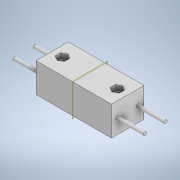
# Autodesk Inventor part: Talon SRX
Saved by Autodesk Inventor 2021 (Build 250183000, 183)
## iProperties
Created: 2021-01-30
Part Number: Talon SRX
Material: Generic
Document SubType Name: Modeling
Designer: aidan
Density: 1 g/cm^3
Appearance: Default
Author: aidan
Autodesk Inventor part; units mm, degrees
ref_plane "YZ Plane" through (0, 0, 0) normal (1, 0, 0) x (0, 1, 0)
ref_plane "XZ Plane" through (0, 0, 0) normal (0, 1, 0) x (-1, 0, 0)
ref_plane "XY Plane" through (0, 0, 0) normal (0, 0, 1) x (1, 0, 0)
sketch "Sketch1" plane through (0, 0, 0) normal (0, 0, 1) x (1, 0, 0)
  line L0 (0, 0) -> (69.85, 0)
  line L1 (69.85, 0) -> (69.85, 27.2034)
  line L2 (69.85, 27.2034) -> (0, 27.2034)
  line L3 (0, 27.2034) -> (0, 0)
  dimension "d0" = 27.2034
  dimension "d1" = 69.85
  constraints: 8 end point, 2 parallel, 1 horizontal, 1 perpendicular
  measures "d0" distance of L0.end L1.end
  measures "d1" distance of L1.end L2.end
extrude "Extrusion1" add sketch "Sketch1" along normal blind 29.9974
sketch "Sketch2" plane through (0, 27.2034, 0) normal (0, 1, 0) x (1, 0, 0)
  line L0 (0, 0) -> (0, -29.9974) projected
  line L1 (0, -15.0114) -> (70.03, -15.0114) construction
  line L2 (69.85, 0) -> (0, 0) projected
  line L3 (9.525, -9.9704) -> (13.8906, -12.4909)
  line L4 (13.8906, -12.4909) -> (13.8906, -17.5319)
  line L5 (13.8906, -17.5319) -> (9.525, -20.0524)
  line L6 (9.525, -20.0524) -> (5.1594, -17.5319)
  line L7 (5.1594, -17.5319) -> (5.1594, -12.4909)
  line L8 (5.1594, -12.4909) -> (9.525, -9.9704)
  line L9 (60.325, -9.9704) -> (64.6906, -12.4909)
  line L10 (64.6906, -12.4909) -> (64.6906, -17.5319)
  line L11 (64.6906, -17.5319) -> (60.325, -20.0524)
  line L12 (60.325, -20.0524) -> (55.9594, -17.5319)
  line L13 (55.9594, -17.5319) -> (55.9594, -12.4909)
  line L14 (55.9594, -12.4909) -> (60.325, -9.9704)
  point P0 (9.525, -15.0114)
  point P1 (60.325, -15.0114)
  dimension "d4" = 15.0114
  dimension "d5" = 50.8
  dimension "d6" = 9.525
  dimension "d7" = 8.7312
  constraints: 26 end point, 3 point on line, 2 vertical, 1 horizontal, 1 parallel, 26 other
  measures "d4" distance between parallel lines of L2 L1
  measures "d5" distance of point (60.325, -15.011) point (9.525, -15.011)
  measures "d6" distance from line of L0 point (9.525, -15.011)
  measures "d7" distance between parallel lines of L7 L4
extrude "Extrusion2" cut sketch "Sketch2" against normal blind 4.5466
sketch "Sketch3" plane through (0, 22.6568, 0) normal (0, 1, 0) x (1, 0, 0)
  line L0 (5.1594, -17.5319) -> (5.1594, -12.4909) projected
  line L1 (9.525, -20.0524) -> (5.1594, -17.5319) projected
  line L2 (13.8906, -17.5319) -> (9.525, -20.0524) projected
  line L3 (13.8906, -12.4909) -> (13.8906, -17.5319) projected
  line L4 (9.525, -9.9704) -> (13.8906, -12.4909) projected
  line L5 (5.1594, -12.4909) -> (9.525, -9.9704) projected
  line L6 (55.9594, -17.5319) -> (55.9594, -12.4909) projected
  line L7 (60.325, -20.0524) -> (55.9594, -17.5319) projected
  line L8 (64.6906, -17.5319) -> (60.325, -20.0524) projected
  line L9 (64.6906, -12.4909) -> (64.6906, -17.5319) projected
  line L10 (60.325, -9.9704) -> (64.6906, -12.4909) projected
  line L11 (55.9594, -12.4909) -> (60.325, -9.9704) projected
  circle A0 centre (9.525, -15.0114) radius 2.2479
  circle A1 centre (60.325, -15.0114) radius 2.2479
  line L12 (5.1594, -15.0114) -> (64.6906, -15.0114) construction
  line L13 (64.6906, -12.4909) -> (64.6906, -17.5319) projected
  line L14 (60.325, -20.0524) -> (60.325, -9.9704) construction
  point P0 (0, 0)
  dimension "d10" = 4.4958
  dimension "d11" = 50.8
  constraints: 4 end point, 3 midpoint, 2 centre point, 2 point on line, 1 equal radius, 1 vertical
  measures "d10" diameter of A0
  measures "d11" distance of A1.centre A0.centre
extrude "Extrusion3" cut sketch "Sketch3" against normal through all contours A0 | A1
sketch "Sketch4" plane through (69.85, 0, 0) normal (1, 0, 0) x (0, 0, -1)
  circle A0 centre (-24.5237, 13.6017) radius 1.5875
  circle A1 centre (-5.4737, 13.6017) radius 1.5875
  line L0 (-29.9974, 27.2034) -> (-29.9974, 0) projected
  line L1 (-29.9974, 13.6017) -> (0, 13.6017) construction
  line L2 (0, 0) -> (0, 27.2034) projected
  line L3 (0, 0) -> (-29.9974, 0) projected
  line L4 (0, 27.2034) -> (-29.9974, 27.2034) projected
  dimension "d14" = 19.05
  dimension "d15" = 27.2034
  dimension "d16" = 13.6017
  dimension "d17" = 3.175
  dimension "d18" = 29.9974
  dimension "d19" = 5.4737
  constraints: 2 centre point, 2 end point, 2 midpoint, 2 point on line, 1 equal radius, 1 horizontal
  measures "d14" distance of A1.centre A0.centre
  measures "d15" distance between parallel lines of L3 L4
  measures "d16" distance between parallel lines of L3 L1
  measures "d17" diameter of A0
  measures "d18" distance of L2.end L0.start
  measures "d19" distance from line of L0 A0.centre
extrude "Extrusion4" add sketch "Sketch4" along normal blind 25.4 contours A0 | A1
ref_plane "Work Plane1" through (34.925, 0, 0) normal (-1, 0, 0) x (0, 0, 1)
mirror "Mirror1" about plane through (34.925, 0, 0) normal (-1, 0, 0) of "Extrusion4"
body "Solid1"
